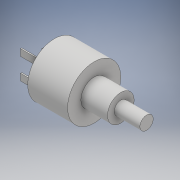
# Autodesk Inventor part: Potentiometer
Saved by Autodesk Inventor 2018 (Build 220112000, 112)
## iProperties
Created: 2019-06-03
Part Number: Potentiometer
Material: Generic
Document SubType Name: Modeling
Designer: aal_9
Density: 1 g/cm^3
Appearance: Default
Author: aal_9
Autodesk Inventor part; units mm, degrees
ref_plane "YZ Plane" through (0, 0, 0) normal (1, 0, 0) x (0, 1, 0)
ref_plane "XZ Plane" through (0, 0, 0) normal (0, 1, 0) x (-1, 0, 0)
ref_plane "XY Plane" through (0, 0, 0) normal (0, 0, 1) x (1, 0, 0)
sketch "Sketch1" plane through (0, 0, 0) normal (1, 0, 0) x (0, 1, 0)
  circle A0 centre (0, 0) radius 6.35
  dimension "d0" = 12.7
  constraints: 1 centre point, 1 coincident
  measures "d0" diameter of A0
extrude "Extrusion1" add sketch "Sketch1" along normal blind 9.5
sketch "Sketch2" plane through (9.5, 0, 0) normal (1, 0, 0) x (0, 0, -1)
  circle A0 centre (0, 0) radius 1.5875
  dimension "d3" = 3.175
  constraints: 1 centre point, 1 coincident
  measures "d3" diameter of A0
extrude "Extrusion2" add sketch "Sketch2" along normal blind 12.5
sketch "Sketch3" plane through (0, 0, 0) normal (-1, 0, 0) x (0, 0, 1)
  line L0 (-0.8, 2.3) -> (0.8, 2.3)
  line L1 (0.8, 2.3) -> (0.8, 2)
  line L2 (0.8, 2) -> (-0.8, 2)
  line L3 (-0.8, 2) -> (-0.8, 2.3)
  line L4 (-3.34, -2.78) -> (-1.74, -2.78)
  line L5 (-1.74, -2.78) -> (-1.74, -3.08)
  line L6 (-1.74, -3.08) -> (-3.34, -3.08)
  line L7 (-3.34, -3.08) -> (-3.34, -2.78)
  line L8 (1.74, -2.78) -> (3.34, -2.78)
  line L9 (3.34, -2.78) -> (3.34, -3.08)
  line L10 (3.34, -3.08) -> (1.74, -3.08)
  line L11 (1.74, -3.08) -> (1.74, -2.78)
  point P0 (0, 0)
  dimension "d6" = 1.6
  dimension "d7" = 0.3
  dimension "d8" = 0.3
  dimension "d9" = 1.6
  dimension "d10" = 1.6
  dimension "d11" = 0.3
  dimension "d12" = 0.8
  dimension "d13" = 2
  dimension "d14" = 4.78
  dimension "d15" = 0
  dimension "d16" = 3.48
  dimension "d17" = 1.74
  constraints: 24 end point, 6 parallel, 3 horizontal, 3 perpendicular
  measures "d6" distance of L0.start L0.end
  measures "d7" distance of L0.end L1.end
  measures "d8" distance of L8.end L9.end
  measures "d9" distance of L9.end L10.end
  measures "d10" distance of L5.end L6.end
  measures "d11" distance of L4.end L5.end
  measures "d12" distance from line of point (0, 0) L3
  measures "d13" distance from line of L2 point (0, 0)
  measures "d14" distance between parallel lines of L8 L2
  measures "d15" distance between parallel lines of L4 L8
  measures "d16" distance between parallel lines of L5 L11
  measures "d17" distance from line of point (0, 0) L5
extrude "Extrusion3" add sketch "Sketch3" along normal blind 5
sketch "Sketch4" plane through (9.5, 0, 0) normal (1, 0, 0) x (0, 0, -1)
  circle A0 centre (0, 0) radius 3.175
  dimension "d20" = 6.35
  constraints: 1 centre point, 1 coincident
  measures "d20" diameter of A0
extrude "Extrusion4" add sketch "Sketch4" along normal blind 6.35
body "Solid1"
